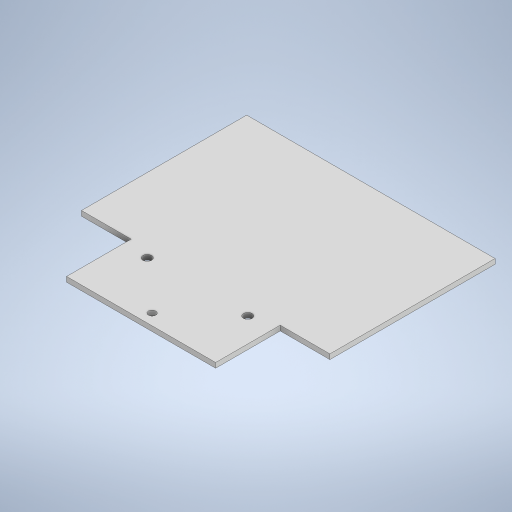
# Autodesk Inventor part: podstawa
Saved by Autodesk Inventor 2023 (Build 270158000, 158)
## iProperties
Created: 2023-07-07
Part Number: podstawa
Material: Ogólny
Document SubType Name: Modeling
Designer: Kamil
Density: 1 g/cm^3
Appearance: Domyślna
Author: Kamil
Autodesk Inventor part; units mm, degrees
ref_plane "YZ Plane" through (0, 0, 0) normal (1, 0, 0) x (0, 1, 0)
ref_plane "XZ Plane" through (0, 0, 0) normal (0, 1, 0) x (-1, 0, 0)
ref_plane "XY Plane" through (0, 0, 0) normal (0, 0, 1) x (1, 0, 0)
sketch "Szkic1" plane through (0, 0, 0) normal (0, 1, 0) x (-1, 0, 0)
  circle A0 centre (45.7688, -11.3479) radius 1.5
  circle A1 centre (25.5188, -29.6192) radius 1.75
  circle A2 centre (66.0188, -29.6192) radius 1.75
  line L0 (-4.2312, -99.4192) -> (95.7688, -99.4192)
  line L1 (95.7688, -99.4192) -> (95.7688, -32.9192)
  line L2 (95.7688, -32.9192) -> (75.7688, -32.9192)
  line L3 (75.7688, -32.9192) -> (75.7688, -6.9192)
  line L4 (75.7688, -6.9192) -> (15.7688, -6.9192)
  line L5 (15.7688, -6.9192) -> (15.7688, -32.9192)
  line L6 (15.7688, -32.9192) -> (-4.2312, -32.9192)
  line L7 (-4.2312, -32.9192) -> (-4.2312, -99.4192)
  point P0 (0, 0)
  point P1 (0, 0)
  constraints: 16 end point, 3 centre point
extrude "Wyciągnięcie proste1" add sketch "Szkic1" along normal blind 2
